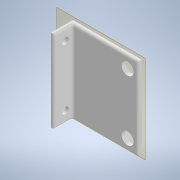
# Autodesk Inventor part: BackPistonSupport Top
Saved by Autodesk Inventor 2022 (Build 260153000, 153)
## iProperties
Created: 2022-02-15
Part Number: BackPistonSupport Top
Material: Generic
Document SubType Name: Modeling
Designer: siwat
Density: 1 g/cm^3
Appearance: Default
VLDS_Profile: Default Part
VLDS_TimeStamp: 2022-03-14
VLDS_FailCnt: 4
VLDS_AcceptCnt: 0
Author: siwat
Autodesk Inventor part; units mm, degrees
ref_plane "YZ Plane" through (0, 0, 0) normal (1, 0, 0) x (0, 1, 0)
ref_plane "XZ Plane" through (0, 0, 0) normal (0, 1, 0) x (-1, 0, 0)
ref_plane "Work Plane1" through (0, 0, 0) normal (0, 0, 1) x (1, 0, 0)
sketch "Sketch1" plane through (0, 0, 0) normal (0, 0, 1) x (1, 0, 0)
  line L0 (-36.5, 37.5) -> (36.5, 37.5)
  arc A0 (37.5, 36.5) -> (36.5, 37.5) centre (36.5, 36.5) ccw
  line L1 (37.5, 36.5) -> (37.5, -36.5)
  line L2 (36.5, -37.5) -> (-36.5, -37.5)
  arc A1 (36.5, -37.5) -> (37.5, -36.5) centre (36.5, -36.5) ccw
  line L3 (37.5, 37.5) -> (-25.4999, 37.5)
  line L4 (-25.4999, 37.5) -> (-25.4999, -37.5)
  line L5 (-25.4999, -37.5) -> (37.5, -37.5)
  line L6 (37.5, -37.5) -> (37.5, 37.5)
  circle A2 centre (27.7, 27.5) radius 5.5
  circle A3 centre (27.7, -27.5) radius 5.5
  point P0 (0, 0)
  point P1 (-25.4999, 37.5)
extrude "Extrusion1" add sketch "Sketch1" along normal blind 3.5 contours L0 A0 L1 A1 L2 L4
sketch "Sketch2" plane through (0, 0, 3.5) normal (0, 0, 1) x (1, 0, 0)
  line L0 (-25.4999, 37.5) -> (-25.4999, -37.5) projected
  line L1 (-25.4999, -37.5) -> (36.5, -37.5) projected
  line L2 (-25.4999, 37.5) -> (-22.4999, 37.5)
  line L3 (-22.4999, 37.5) -> (-22.4999, -37.5)
  line L4 (-22.4999, -37.5) -> (-25.4999, -37.5)
  line L5 (-25.4999, -37.5) -> (-25.4999, 37.5)
  point P0 (0, 0)
  dimension "d2" = 3
  constraints: 8 end point, 2 parallel, 1 horizontal, 1 perpendicular, 1 point on line
  measures "d2" distance of L3.end L4.end
ref_plane "Work Plane2" through (-30.7961, -197.5, 20) normal (0, 0, 1) x (1, 0, 0)
extrude "Extrusion2" add sketch "Sketch2" along normal blind 16.5
sketch "Sketch3" plane through (-22.4999, -37.5, 3.5) normal (1, 0, 0) x (0, 0, -1)
  circle A0 centre (-6.5, 65) radius 3
  circle A1 centre (-6.5, 10) radius 3
  line L0 (-6.5, 10) -> (-6.5, 65)
  line L1 (0, 75) -> (-16.5, 75) projected
  line L2 (0, 0) -> (-16.5, 0) projected
  line L3 (-16.5, 0) -> (-16.5, 75) projected
  point P0 (3.5, 37.5)
  point P1 (-6.5, 37.5)
  dimension "d5" = 6
  dimension "d6" = 6
  dimension "d7" = 10
  dimension "d8" = 10
  dimension "d9" = 10
  constraints: 2 centre point, 2 end point, 1 midpoint, 1 vertical
  measures "d5" diameter of A0
  measures "d6" diameter of A1
  measures "d7" distance from line of L0.end L1
  measures "d8" distance from line of L2 L0.start
  measures "d9" distance from line of L3 point (-6.5, 37.5)
extrude "Extrusion3" cut sketch "Sketch3" against normal blind 16.5
body "Solid1"
